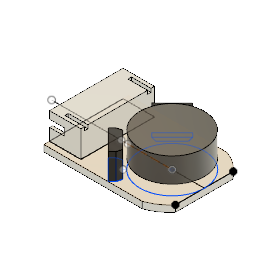
4afd0742-d21b-4b30-ba88-0911411fe08a (Autodesk Fusion 360 design; units mm, degrees)
Autodesk Fusion 360 part; units mm, degrees
sketch "Sketch1" plane through (0, 0, 0) normal (0, 1, 0) x (1, 0, 0)
  line L0 (2.8257, 4.125) -> (2.8257, -4.125)
  line L1 (0, 0) -> (0, 6.05)
  line L2 (0, 0) -> (0, -5)
  line L3 (0, 0) -> (0, -6.05)
  arc A0 (2.8257, 4.125) -> (0, 6.05) centre (-2.0531, 0) ccw
  arc A1 (0, -6.05) -> (2.8257, -4.125) centre (-2.0531, 0) ccw
  line L4 (2.8257, 0) -> (-14.0343, 0)
  line L5 (-14.0343, 0) -> (-14.0343, 6.05)
  line L6 (-14.0343, 0) -> (-14.0343, -6.05)
  line L7 (0, 6.05) -> (-14.0343, 6.05)
  line L8 (-14.0343, 6.05) -> (-14.0343, -6.05)
  line L9 (-14.0343, -6.05) -> (0, -6.05)
  line L10 (0, -6.05) -> (0, 6.05)
  dimension "d2" = 8.25
  dimension "d6" = 16.86
  dimension "d7" = 6.05
  dimension "d8" = 6.05
  constraint vertical L0
  constraint vertical L1
  constraint parallel L1 L2
  constraint parallel L2 L3
  constraint coincident L3.end A0
  constraint concentric A0 A1
  constraint midpoint L0 L4.start
  constraint perpendicular L0 L4
  constraint perpendicular L4 L5
  constraint perpendicular L4 L6
  constraint perpendicular L7 L8
  constraint parallel L7 L9
  constraint parallel L8 L10
  constraint perpendicular L5 L7
  measures "d2" distance of L0.start L0.end
  measures "d6" distance of L4.start L4.end
  measures "d7" distance of L4.end L5.end
  measures "d8" distance of L4.end L6.end
extrude "Extrude1" add sketch "Sketch1" along normal blind 0.94 makes body 1
sketch "Sketch3" plane through (0, 0.94, 0) normal (0, 1, 0) x (-1, 0, 0)
  arc A0 (-2.8257, -4.125) -> (0, -6.05) centre (2.0531, 0) ccw
  line L0 (0, -6.05) -> (14.0343, -6.05)
  line L1 (14.0343, -6.05) -> (14.0343, 6.05)
  line L2 (14.0343, 6.05) -> (0, 6.05)
  arc A1 (0, 6.05) -> (-2.8257, 4.125) centre (2.0531, 0) ccw
  line L3 (-2.8257, 4.125) -> (-2.8257, -4.125)
  line L4 (-2.8257, -4.125) -> (-2.8257, 4.125)
  line L5 (-2.8257, 0) -> (6.3443, 0)
  circle A2 centre (1.7593, 0) radius 4.585
  circle A3 centre (1.7593, 0) radius 0.25
  line L6 (14.0343, 0) -> (14.0343, -5.25)
  line L7 (14.0343, 0) -> (14.0343, 5.25)
  line L8 (14.0343, -5.25) -> (14.0343, 5.25)
  line L9 (14.0343, 5.25) -> (9.5343, 5.25)
  line L10 (9.5343, 5.25) -> (9.5343, -5.25)
  line L11 (9.5343, -5.25) -> (14.0343, -5.25)
  line L12 (6.3443, 0) -> (18.9648, 0)
  line L13 (1.7593, 0) -> (9.0593, 0) construction
  line L14 (1.7593, 0) -> (8.0593, 0) construction
  line L15 (6.3202, 4.5608) -> (4.8529, 6.0281)
  line L16 (6.3202, 4.5608) -> (7.7874, 3.0936)
  line L17 (4.8529, 6.0281) -> (7.7874, 3.0936)
  line L18 (7.7874, 3.0936) -> (7.2429, 2.5491)
  line L19 (7.2429, 2.5491) -> (4.3085, 5.4836)
  line L20 (4.3085, 5.4836) -> (4.8529, 6.0281)
  line L21 (6.4651, 2.337) -> (4.0963, 4.7058)
  line L22 (4.0963, 4.7058) -> (4.3085, 5.4836)
  line L23 (6.4651, 2.337) -> (7.2429, 2.5491)
  line L24 (1.7593, 0) -> (1.9361, 0.1768)
  line L25 (5.0014, 3.2421) -> (5.2807, 3.5214)
  line L26 (6.4651, -2.337) -> (4.0963, -4.7058)
  line L27 (6.4651, -2.337) -> (7.2429, -2.5491)
  line L28 (7.7874, -3.0936) -> (7.2429, -2.5491)
  line L29 (4.8529, -6.0281) -> (7.7874, -3.0936)
  line L30 (4.3085, -5.4836) -> (4.8529, -6.0281)
  line L31 (4.0963, -4.7058) -> (4.3085, -5.4836)
  line L32 (7.2429, -2.5491) -> (4.3085, -5.4836)
  dimension "d16" = 0.5
  dimension "d19" = 5.25
  dimension "d20" = 5.25
  dimension "d21" = 4.5
  constraint coincident A0.start L3.end
  constraint coincident A1.end L3.start
  constraint midpoint L3 L5.start
  constraint perpendicular L4 L5
  constraint coincident L5.start A2
  constraint tangent L4 A2
  constraint coincident L5.end A2
  constraint concentric A2 A3
  constraint midpoint L1 L6.start
  constraint parallel L1 L6
  constraint parallel L1 L7
  constraint perpendicular L8 L9
  constraint parallel L8 L10
  constraint parallel L9 L11
  constraint perpendicular L10 L12
  constraint horizontal L13
  constraint coincident A2.centre A3.centre
  constraint horizontal L14
  constraint perpendicular L15 L24
  constraint perpendicular L16 L24
  constraint perpendicular L17 L18
  constraint parallel L17 L19
  constraint parallel L18 L20
  constraint perpendicular L21 L24
  constraint coincident L21 L25.end
  constraint coincident A3 L24.end
  constraint coincident A2 L25.start
  constraint collinear L24 L25
  constraint symmetric L12 L15.end L29.start
  constraint symmetric L12 L16.end L28.start
  constraint symmetric L12 L18.end L27.end
  constraint symmetric L12 L19.end L30.start
  constraint symmetric L12 L21.start L26.start
  constraint symmetric L12 L21.end L26.end
  measures "d16" diameter of A3
  measures "d19" distance of L6.start L6.end
  measures "d20" distance of L6.start L7.end
  measures "d21" distance of L6.end L10.end
extrude "Extrude10" add sketch "Sketch3" along normal blind 3.7 contours L15 L16 L17 L18 L19 L20 | L19 L21 L22 L23 | L26 L27 L31 L32 | L28 L29 L30 L32 bodies 1
extrude "Extrude5" add sketch "Sketch3" along normal blind 3.79 contours L1 L6 L8 L10 L11 L12 | L1 L7 L8 L9 L10 L12 bodies 1
extrude "Extrude4" add sketch "Sketch3" along normal blind 1.42 separate body contours L5 A3 L24 | L5 A3 | L5 A3 L24 makes body 2
extrude "Extrude2" add sketch "Sketch3" along normal blind 4.93 contours L5 A2 A3 | L5 A2 A3 | L5 A3 L24 | L5 A3 | L5 A3 L24 bodies 1
sketch "Sketch5" plane through (0, 0.94, 0) normal (0, 1, 0) x (-1, 0, 0)
  arc A0 (-2.8257, -4.125) -> (0, -6.05) centre (2.0531, 0) ccw
  line L0 (0, -6.05) -> (14.0343, -6.05)
  line L1 (14.0343, 5.25) -> (14.0343, 6.05)
  line L2 (14.0343, 6.05) -> (0, 6.05)
  arc A1 (0, 6.05) -> (-2.8257, 4.125) centre (2.0531, 0) ccw
  line L3 (-2.8257, 4.125) -> (-2.8257, 0)
  circle A2 centre (1.7593, 0) radius 4.585
  line L4 (-2.8257, 0) -> (-2.8257, -4.125)
  circle A3 centre (1.7593, 0) radius 4.585
  line L5 (9.5343, 5.25) -> (14.0343, 5.25)
  line L6 (14.0343, -6.05) -> (14.0343, -5.25)
  line L7 (14.0343, -5.25) -> (9.5343, -5.25)
  line L8 (9.5343, -5.25) -> (9.5343, 5.25)
  line L9 (6.4651, -2.337) -> (7.2429, -2.5491)
  line L10 (7.2429, -2.5491) -> (7.7874, -3.0936)
  line L11 (7.7874, -3.0936) -> (4.8529, -6.0281)
  line L12 (4.8529, -6.0281) -> (4.3085, -5.4836)
  line L13 (4.3085, -5.4836) -> (4.0963, -4.7058)
  line L14 (4.0963, -4.7058) -> (6.4651, -2.337)
  line L15 (4.0963, 4.7058) -> (4.3085, 5.4836)
  line L16 (4.3085, 5.4836) -> (4.8529, 6.0281)
  line L17 (4.8529, 6.0281) -> (7.7874, 3.0936)
  line L18 (7.7874, 3.0936) -> (7.2429, 2.5491)
  line L19 (7.2429, 2.5491) -> (6.4651, 2.337)
  line L20 (6.4651, 2.337) -> (4.0963, 4.7058)
  constraint concentric A2 A3
extrude "Extrude3" cut sketch "Sketch5" along normal blind 1.42 contours A2 A3 bodies 1 makes body 3 at (-9.3562, 0, -2.0167)
sketch "Sketch6" plane through (-14.0343, 0, 0) normal (-1, 0, 0) x (0, 0, 1)
  line L0 (-6.05, 0) -> (6.05, 0)
  line L1 (6.05, 0) -> (6.05, 0.94)
  line L2 (6.05, 0.94) -> (5.25, 0.94)
  line L3 (5.25, 0.94) -> (5.25, 4.73)
  line L4 (5.25, 4.73) -> (-5.25, 4.73)
  line L5 (-5.25, 4.73) -> (-5.25, 0.94)
  line L6 (-5.25, 0.94) -> (-6.05, 0.94)
  line L7 (-6.05, 0.94) -> (-6.05, 0)
  line L8 (0, 0) -> (0, 0.94)
  line L9 (0, 0.94) -> (-4.81, 0.94)
  line L10 (0, 0.94) -> (4.81, 0.94)
  line L11 (0, 0) -> (0, 6.2135)
  line L12 (0, 0.94) -> (0, 1.34)
  line L13 (0, 4.73) -> (0, 4.18)
  line L14 (4.81, 0.94) -> (4.81, 4.73)
  line L15 (0, 4.18) -> (5.25, 4.18)
  line L16 (4.81, 4.18) -> (4.81, 0.94)
  line L17 (4.81, 0.94) -> (-4.81, 0.94)
  line L18 (-4.81, 0.94) -> (-4.81, 4.18)
  line L19 (-4.81, 4.18) -> (4.81, 4.18)
  dimension "d24" = 0.94
  dimension "d25" = 4.81
  dimension "d26" = 4.81
  dimension "d27" = 0.4
  dimension "d28" = 0.55
  constraint coincident L8.start L11.start
  constraint perpendicular L0 L8
  constraint perpendicular L8 L9
  constraint perpendicular L8 L10
  constraint perpendicular L0 L11
  constraint perpendicular L9 L12
  constraint midpoint L4 L13.start
  constraint perpendicular L4 L13
  constraint coincident L4 L14.end
  constraint perpendicular L4 L14
  constraint coincident L3 L15.end
  constraint perpendicular L3 L15
  constraint perpendicular L16 L17
  constraint parallel L16 L18
  constraint parallel L17 L19
  constraint perpendicular L10 L16
  constraint coincident L15 L16.start
  measures "d24" distance of L8.start L8.end
  measures "d25" distance of L8.end L9.end
  measures "d26" distance of L8.end L10.end
  measures "d27" distance of L8.end L12.end
  measures "d28" distance of L13.start L13.end
extrude "Extrude6" cut sketch "Sketch6" against normal blind 2.4 contours L10 L11 L12 L14 L15 L16 L17 L19 | L9 L11 L12 L17 L18 L19 bodies 3
sketch "Sketch7" plane through (0, 0, -5.25) normal (0, 0, -1) x (-1, 0, 0)
  line L0 (9.5343, 0.94) -> (14.0343, 0.94)
  line L1 (14.0343, 0.94) -> (14.0343, 4.73)
  line L2 (14.0343, 4.73) -> (9.5343, 4.73)
  line L3 (9.5343, 4.73) -> (9.5343, 0.94)
  line L4 (14.0343, 4.73) -> (14.0343, 3.65)
  line L5 (14.0343, 3.65) -> (14.0343, 2.66)
  line L6 (14.0343, 3.65) -> (12.0343, 3.65)
  line L7 (12.0343, 3.65) -> (12.0343, 2.66)
  line L8 (12.0343, 2.66) -> (14.0343, 2.66)
  line L9 (14.0343, 2.66) -> (14.0343, 3.65)
  dimension "d31" = 1.08
  dimension "d32" = 0.99
  dimension "d33" = 2
  constraint coincident L1.end L2.start
  constraint perpendicular L2 L4
  constraint coincident L1 L5.end
  constraint horizontal L6
  constraint vertical L7
  constraint horizontal L8
  constraint vertical L9
  measures "d31" distance of L1.end L4.end
  measures "d32" distance of L4.end L5.end
  measures "d33" distance of L4.end L6.end
extrude "Extrude7" cut sketch "Sketch7" against normal blind 0.44 contours L1 L5 L6 L7 L8 L9 bodies 3
sketch "Sketch8" plane through (0, 0, 5.25) normal (0, 0, 1) x (1, 0, 0)
  line L0 (-14.0343, 0.94) -> (-9.5343, 0.94)
  line L1 (-9.5343, 0.94) -> (-9.5343, 4.73)
  line L2 (-9.5343, 4.73) -> (-14.0343, 4.73)
  line L3 (-14.0343, 4.73) -> (-14.0343, 0.94)
  line L4 (-14.0343, 4.73) -> (-14.0343, 3.65)
  line L5 (-14.0343, 3.65) -> (-14.0343, 2.66)
  line L6 (-14.0343, 3.65) -> (-11.9343, 3.65)
  line L7 (-11.9343, 3.65) -> (-11.9343, 2.66)
  line L8 (-11.9343, 2.66) -> (-14.0343, 2.66)
  line L9 (-14.0343, 2.66) -> (-14.0343, 3.65)
  dimension "d36" = 1.08
  dimension "d37" = 0.99
  dimension "d38" = 2.1
  constraint coincident L2.end L3.start
  constraint perpendicular L2 L4
  constraint perpendicular L0 L5
  constraint horizontal L6
  constraint vertical L7
  constraint horizontal L8
  constraint vertical L9
  measures "d36" distance of L2.end L4.end
  measures "d37" distance of L4.end L5.end
  measures "d38" distance of L4.end L6.end
extrude "Extrude8" cut sketch "Sketch8" against normal blind 0.44 contours L3 L5 L6 L7 L8 L9 bodies 3
sketch "Sketch9" plane through (0, 4.73, 0) normal (0, 1, 0) x (-1, 0, 0)
  line L0 (9.5343, -5.25) -> (14.0343, -5.25)
  line L1 (14.0343, -5.25) -> (14.0343, 5.25)
  line L2 (14.0343, 5.25) -> (9.5343, 5.25)
  line L3 (9.5343, 5.25) -> (9.5343, -5.25)
  line L4 (9.5343, -5.25) -> (9.5343, -4.75)
  line L5 (14.0343, 0) -> (9.5343, 0)
  line L6 (9.5343, -4.75) -> (9.5343, -4.25)
  line L7 (9.5343, -4.75) -> (9.5343, -4.25)
  line L8 (9.5343, -4.25) -> (12.3343, -4.25)
  line L9 (12.3343, -4.25) -> (12.3343, -4.75)
  line L10 (12.3343, -4.75) -> (9.5343, -4.75)
  line L11 (12.3343, 4.75) -> (9.5343, 4.75)
  line L12 (9.5343, 4.25) -> (12.3343, 4.25)
  line L13 (12.3343, 4.25) -> (12.3343, 4.75)
  line L14 (9.5343, 4.75) -> (9.5343, 4.25)
  dimension "d41" = 0.5
  dimension "d42" = 0.5
  dimension "d43" = 2.8
  constraint coincident L0.start L3.end
  constraint perpendicular L0 L4
  constraint midpoint L1 L5.start
  constraint midpoint L3 L5.end
  constraint perpendicular L5 L6
  constraint perpendicular L7 L8
  constraint parallel L7 L9
  constraint parallel L8 L10
  constraint parallel L6 L7
  constraint symmetric L4.end L5 L11.end
  constraint symmetric L5 L6.end L12.start
  constraint symmetric L5 L8.end L12.end
  constraint symmetric L5 L9.end L11.start
  measures "d41" distance of L0.start L4.end
  measures "d42" distance of L4.end L6.end
  measures "d43" distance of L4.end L9.end
extrude "Extrude9" cut sketch "Sketch9" against normal blind 0.5 contours L3 L6 L7 L8 L9 L10 | L3 L11 L12 L13 L14 bodies 3
